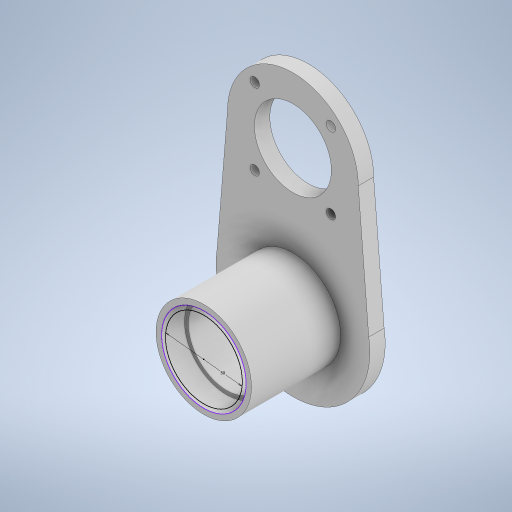
# Autodesk Inventor part: podstwa_obrotowa
Saved by Autodesk Inventor 2023 (Build 270158000, 158)
## iProperties
Created: 2023-03-28
Part Number: podstwa_obrotowa
Material: Ogólny
Document SubType Name: Modeling
Designer: krzys
Density: 1 g/cm^3
Appearance: Domyślna
Author: krzys
Autodesk Inventor part; units mm, degrees
ref_plane "YZ Plane" through (0, 0, 0) normal (1, 0, 0) x (0, 1, 0)
ref_plane "XZ Plane" through (0, 0, 0) normal (0, 1, 0) x (-1, 0, 0)
ref_plane "XY Plane" through (0, 0, 0) normal (0, 0, 1) x (1, 0, 0)
sketch "Szkic1" plane through (0, 0, 0) normal (0, 0, 1) x (1, 0, 0)
  circle A0 centre (0, 0) radius 27.5
  circle A1 centre (0, 0) radius 31
  arc A2 (-49.3103, 8.2759) -> (49.3103, 8.2759) centre (0, 0) ccw
  circle A3 centre (0, 90) radius 25
  arc A4 (42.5, 90) -> (-42.5, 90) centre (0, 90) ccw
  circle A5 centre (24.7487, 65.2513) radius 3
  circle A6 centre (24.7487, 114.7487) radius 3
  circle A7 centre (-24.7487, 114.7487) radius 3
  circle A8 centre (-24.7487, 65.2513) radius 3
  line L0 (-42.5, 90) -> (-49.3103, 8.2759)
  line L1 (42.5, 90) -> (49.3103, 8.2759)
  circle A9 centre (0, 0) radius 25
  dimension "d0" = 55
  dimension "d1" = 62
  dimension "d2" = 100
  dimension "d3" = 50
  dimension "d4" = 85
  dimension "d5" = 6
  dimension "d8" = 360
  dimension "d10" = 50
  constraints: 10 centre point, 5 coincident, 4 end point, 4 point on circle, 1 other
  measures "d0" diameter of A0
  measures "d1" diameter of A1
  measures "d2" diameter of A2
  measures "d3" diameter of A3
  measures "d4" diameter of A4
  measures "d5" diameter of A5
  measures "d10" diameter of A9
extrude "Wyciągnięcie proste1" add sketch "Szkic1" along normal blind 68 contours A1
extrude "Wyciągnięcie proste2" add sketch "Szkic1" along normal blind 10 contours L0 A4 L1 A2
sketch "Szkic2" plane through (0, 0, 68) normal (0, 0, 1) x (1, 0, 0)
  circle A0 centre (0, 0) radius 25
  circle A1 centre (0, 0) radius 27.4549
  dimension "d15" = 50
  constraints: 2 centre point, 1 coincident
  measures "d15" diameter of A0
extrude "Wyciągnięcie proste3" add sketch "Szkic2" against normal blind 50
extrude "Wyciągnięcie proste5" cut sketch "Szkic2" against normal blind 15
